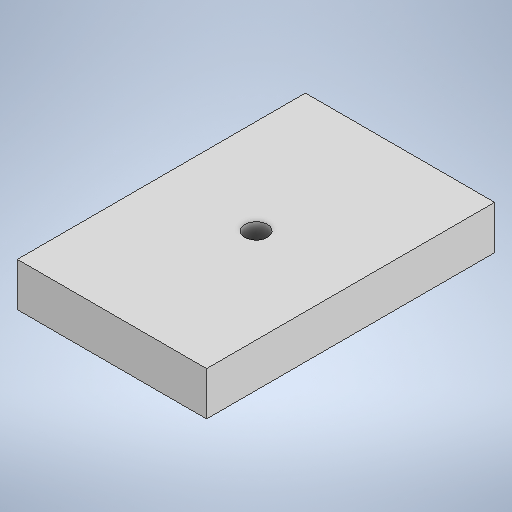
# Autodesk Inventor part: servoArm
Saved by Autodesk Inventor 2025.1 (Build 291241020, 241B)
## iProperties
Created: 2024-09-10
Part Number: servoArm
Material: Generic
Document SubType Name: Modeling
Designer: omiye
Density: 1 g/cm^3
Appearance: Default
Author: omiye
Autodesk Inventor part; units mm, degrees
ref_plane "YZ Plane" through (0, 0, 0) normal (1, 0, 0) x (0, 1, 0)
ref_plane "XZ Plane" through (0, 0, 0) normal (0, 1, 0) x (-1, 0, 0)
ref_plane "XY Plane" through (0, 0, 0) normal (0, 0, 1) x (1, 0, 0)
sketch "Sketch1" plane through (0, 0, 0) normal (1, 0, 0) x (0, 1, 0)
  line L0 (2.875, -19) -> (-2.875, -19)
  line L1 (-2.875, -19) -> (-2.875, 19)
  line L2 (-2.875, 19) -> (2.875, 19)
  line L3 (2.875, 19) -> (2.875, -19)
  line L4 (2.875, -19) -> (-2.875, 19) construction
  line L5 (-2.875, -19) -> (2.875, 19) construction
  point P0 (0, 0)
  dimension "d0" = 5.75
  dimension "d1" = 38
  constraints: 12 end point, 2 midpoint, 2 parallel, 1 horizontal, 1 perpendicular
  measures "d0" distance of L1.end L2.end
  measures "d1" distance of L0.end L1.end
extrude "Extrusion1" add sketch "Sketch1" along normal blind 12.5
sketch "Sketch2" plane through (0, 2.875, 19) normal (0, 1, 0) x (1, 0, 0)
  circle A0 centre (6.25, 19) radius 1.5
  point P0 (0, 19)
  dimension "d4" = 3
  constraints: 1 centre point
  measures "d4" diameter of A0
extrude "Extrusion2" cut sketch "Sketch2" against normal blind 12.5
sketch "Sketch3" plane through (12.5, 0, 0) normal (1, 0, 0) x (0, 0, -1)
  point P0 (0, 0)
sketch "Sketch4" plane through (0, -2.875, -19) normal (0, -1, 0) x (1, 0, 0)
  line L0 (0, 0) -> (0, 38) projected
  line L1 (0, 0) -> (-6.25, 0)
  line L2 (-6.25, 0) -> (-6.25, 38)
  line L3 (-6.25, 38) -> (0, 38)
  line L4 (0, 38) -> (0, 0)
  line L5 (12.4682, 38) -> (18.7182, 38)
  line L6 (18.7182, 38) -> (18.7182, 0)
  line L7 (18.7182, 0) -> (12.4682, 0)
  line L8 (12.4682, 0) -> (12.4682, 38)
  point P0 (0, 19)
  dimension "d7" = 6.25
  dimension "d8" = 6.25
  constraints: 16 end point, 4 parallel, 2 horizontal, 2 perpendicular, 2 point on line
  measures "d7" distance of L2.end L3.end
  measures "d8" distance of L6.end L7.end
extrude "Extrusion3" add sketch "Sketch4" against normal up to surface (5.75 mm away)
body "Solid1"
